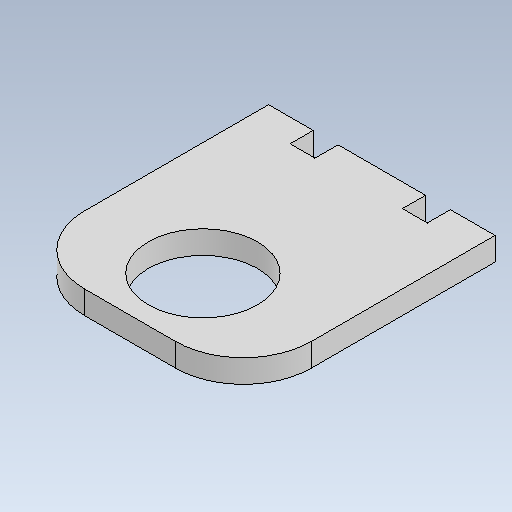
# Autodesk Inventor part: motorholder1A
Saved by Autodesk Inventor 2025 (Build 290162000, 162)
## iProperties
Created: 2024-08-15
Part Number: motorholder1A
Material: Polycarbonate, Smoke
Document SubType Name: Modeling
Designer: PC
Density: 1.2 g/cm^3
Appearance: Default
Author: PC
Autodesk Inventor part; units mm, degrees
ref_plane "YZ Plane" through (0, 0, 0) normal (1, 0, 0) x (0, 1, 0)
ref_plane "XZ Plane" through (0, 0, 0) normal (0, 1, 0) x (-1, 0, 0)
ref_plane "XY Plane" through (0, 0, 0) normal (0, 0, 1) x (1, 0, 0)
sketch "Sketch1" plane through (0, 0, 0) normal (0, 0, 1) x (1, 0, 0)
  line L0 (25, -2.55) -> (-25, -2.55)
  line L1 (-25, -2.55) -> (-25, 2.55)
  line L2 (-25, 2.55) -> (25, 2.55)
  line L3 (25, 2.55) -> (25, -2.55)
  line L4 (25, -2.55) -> (-25, 2.55) construction
  line L5 (-25, -2.55) -> (25, 2.55) construction
  point P0 (0, 0)
  dimension "d0" = 50
  dimension "d1" = 5.1
  constraints: 12 end point, 2 midpoint, 2 parallel, 1 horizontal, 1 perpendicular
  measures "d0" distance of L1.end L2.end
  measures "d1" distance of L0.end L1.end
extrude "Extrusion1" add sketch "Sketch1" along normal blind 45.1
sketch "Sketch2" plane through (-25, -2.55, 0) normal (0, -1, 0) x (1, 0, 0)
  line L0 (50, 0) -> (0, 0) projected
  line L1 (9.85, 0) -> (15.35, 0)
  line L2 (15.35, 0) -> (15.35, 5.1)
  line L3 (15.35, 5.1) -> (9.85, 5.1)
  line L4 (9.85, 5.1) -> (9.85, 0)
  line L5 (40.15, 0) -> (34.65, 0)
  line L6 (34.65, 0) -> (34.65, 5.1)
  line L7 (34.65, 5.1) -> (40.15, 5.1)
  line L8 (40.15, 5.1) -> (40.15, 0)
  line L9 (50, 0) -> (50, 45.1) projected
  line L10 (0, 0) -> (0, 45.1) projected
  point P0 (25, 0)
  point P1 (40.15, 2.55)
  dimension "d5" = 5.1
  dimension "d9" = 5.1
  dimension "d17" = 9.85
  dimension "d25" = 5.5
  dimension "d26" = 5.5
  dimension "d27" = 9.85
  constraints: 16 end point, 4 parallel, 2 horizontal, 2 perpendicular, 2 point on line, 1 midpoint
  measures "d5" distance of L2.end L1.end
  measures "d9" distance of L5.start L7.end
  measures "d17" distance from line of L9 point (40.15, 2.55)
  measures "d25" distance between parallel lines of L6 L8
  measures "d26" distance between parallel lines of L2 L4
  measures "d27" distance between parallel lines of L10 L4
extrude "Extrusion2" cut sketch "Sketch2" against normal blind 45.1
sketch "Sketch3" plane through (-25, -2.55, 45.1) normal (0, -1, 0) x (1, 0, 0)
  circle A0 centre (25, -5.6) radius 3.45
  line L0 (0, 0) -> (50, 0) projected
  circle A1 centre (25, -5.6) radius 12.05
  line L1 (50, 0) -> (0, 0)
  line L2 (0, 0) -> (0, 10.45)
  line L3 (0, 10.45) -> (50, 10.45)
  line L4 (50, 10.45) -> (50, 0)
  line L5 (0, -45.1) -> (0, 0) projected
  point P0 (25, -45.1)
  point P1 (14.3303, 0)
  point P2 (35.6697, 0)
  dimension "d12" = 6.9
  dimension "d13" = 5.6
  dimension "d14" = 25
  dimension "d19" = 24.1
  dimension "d20" = 16.05
  constraints: 8 end point, 2 centre point, 2 parallel, 1 coincident, 1 collinear, 1 horizontal, 1 perpendicular
  measures "d12" diameter of A0
  measures "d13" distance from line of L0 A0.centre
  measures "d14" horizontal distance of L0.start A0.centre
  measures "d19" diameter of A1
  measures "d20" distance from line of L3 A1.centre
extrude "Extrusion3" cut sketch "Sketch3" against normal blind 45.1 contours A0 | L0 A1 picked at (25.1386, -0.7251)
extrude "Extrusion4" add sketch "Sketch3" against normal up to surface (5.1 mm away) contours L2 L3 L4 L0 A1
fillet "Fillet1" radius 15 2 edges at (25, 0, 55.55) (-25, 0, 55.55)
equation "\"d26\" = d25"
equation "\"d27\" = d17"
body "Solid1"
